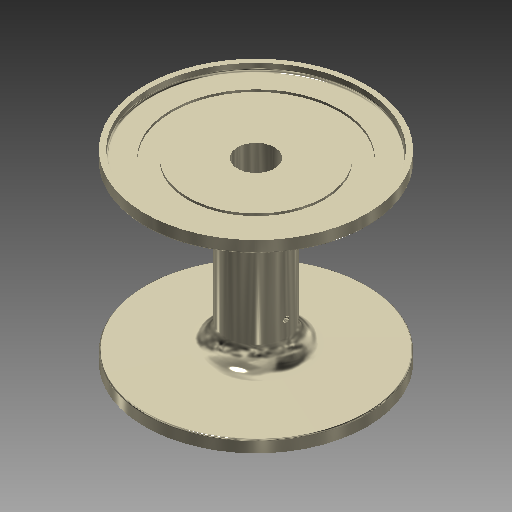
# Autodesk Inventor part: 402-01
Saved by Autodesk Inventor 2019 (Build 230136000, 136)
## iProperties
Company: Autodesk Inc.
Created: 2017-06-27
Part Number: 402-01
Material: PAEK Plastic
Document SubType Name: Modeling
Designer: Autodesk Inc.
Mass: 6.33082 g
Surface Area: 67.4982 cm^2
Volume: 4.79608 cm^3
Density: 1.32 g/cm^3
Appearance: Nickel
Author: Inventor
Autodesk Inventor part; units mm, degrees
ref_plane "XZ Plane" through (0, 0, 0) normal (0, 1, 0) x (-1, 0, 0)
ref_plane "XY Plane" through (0, 0, 0) normal (0, 0, 1) x (1, 0, 0)
sketch "Sketch1" plane through (0, 0, 0) normal (0, 0, 1) x (1, 0, 0)
  line L0 (0, 0) -> (5.3, 0)
  line L1 (0, 14.9) -> (0, 0)
  line L2 (0, 14.9) -> (11.95, 14.9)
  line L3 (11.95, 14.9) -> (14.75, 14.9)
  line L4 (14.75, 14.9) -> (14.75, 14.5)
  line L5 (14.75, 14.5) -> (11.95, 14.5)
  line L6 (11.95, 14.5) -> (11.95, 14.9)
  line L7 (14.75, 14.9) -> (18.6, 14.9)
  line L8 (18.6, 14.9) -> (18.6, 16.2)
  line L9 (18.6, 16.2) -> (19.5, 16.2)
  line L10 (19.5, 16.2) -> (19.5, 14.4)
  line L11 (19.2255, 14.1011) -> (8.5028, 13.1874)
  line L12 (5.3, 9.7) -> (5.3, 0)
  arc A0 (19.2255, 14.1011) -> (19.5, 14.4) centre (19.2, 14.4) ccw
  arc A1 (8.5028, 13.1874) -> (5.3, 9.7) centre (8.8, 9.7) ccw
  dimension "d0" = 32.4
  dimension "d2" = 1.3
  dimension "d3" = 1.7
  dimension "d4" = 23.9
  dimension "d5" = 39
  dimension "d6" = 37.2
  dimension "d7" = 10.6
  dimension "d8" = 2.8
  dimension "d9" = 0.3
  dimension "d10" = 3.5
  dimension "d11" = 1.8
  dimension "d12" = 6.5
  constraints: 26 end point, 5 parallel, 4 perpendicular, 4 point on circle, 4 tangent, 2 centre point, 2 horizontal
  measures "d0" diameter of L9 L0
  measures "d2" distance between parallel lines of L9 L7
  measures "d3" distance between parallel lines of L5 L9
  measures "d4" diameter of L6 L1
  measures "d5" diameter of L10 L1
  measures "d6" diameter of L8 L1
  measures "d7" diameter of L12 L1
  measures "d8" distance of L2.end L3.end
  measures "d9" radius of A0
  measures "d10" radius of A1
  measures "d11" distance from line of A0.centre L9
  measures "d12" distance from line of A1.centre L9
revolve "Revolution1" add sketch "Sketch1" angle 360 about axis through (0, 14.9, 0) along (0, -1, 0)
mirror "Mirror1" about plane through (2.65, 0, 0) normal (0, -1, 0)
hole "Hole1" at (0, 14.9, 0) direction (0, -1, 0) diameter 6.5 end through all
revolve "Revolution2" cut sketch "Sketch1" angle 360 about axis through (0, 14.9, 0) along (0, -1, 0) contours L3 L4 L5 L6
fillet "Fillet1" radius 0.5 2 edges at (-18.6, 14.9, 0) (-18.6, -14.9, 0)
ref_plane "Work Plane1" through (-5.3, 4.85, 0) normal (1, 0, 0) x (0, 1, 0)
sketch "Sketch3" plane through (-5.3, 4.85, 0) normal (1, 0, 0) x (0, 1, 0)
  point P0 (-4.85, 0)
  point P1 (-11.85, 0)
  dimension "d35" = 7
  constraints: 1 horizontal alignment
  measures "d35" distance of point (-11.85, 0) point (-4.85, 0)
hole "Hole2" at (-5.3, -7, 0) direction (1, 0, 0) diameter 0.5 end through all countersink diameter 1 countersink angle 50
ref_plane "Work Plane2" through (5.3, 4.85, 0) normal (1, 0, 0) x (0, 1, 0)
hole "Hole3" at (5.3, -7, 0) direction (-1, 0, 0) diameter 0.5 depth 1 tip angle 118 countersink diameter 1 countersink angle 50
body "Solid1"
